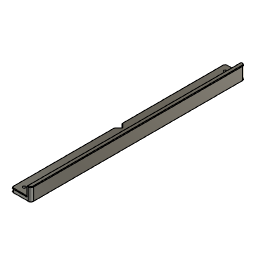
bed_hole_marking_template_x1_Rev2 (Autodesk Fusion 360 design; units mm, degrees)
Autodesk Fusion 360 part; units mm, degrees
sketch "Sketch1" plane through (0, 0, 0) normal (0, 0, 1) x (1, 0, 0) in component "bed_hole_marking_template_x1_Rev2"
  line L0 (7.5, -80) -> (-7.5, -80)
  line L1 (-7.5, -80) -> (-7.5, 80)
  line L2 (-7.5, 80) -> (7.5, 80)
  line L3 (7.5, 80) -> (7.5, -80)
  line L4 (7.5, -80) -> (-7.5, 80) construction
  line L5 (-7.5, -80) -> (7.5, 80) construction
  line L6 (-4.5, -0.0061) -> (-7.5, 2.9939)
  line L7 (0, 0) -> (-10, 0) construction
  circle A0 centre (-2.5, 75) radius 1
  line L8 (-4.5, 0.0061) -> (-7.5, -2.9939)
  line L9 (4.5, 80) -> (4.5, -80)
  circle A1 centre (-2.5, -75) radius 1
  point P0 (-2.5, -75)
  dimension "d1" = 15
  dimension "d2" = 160
  dimension "d3" = 135
  dimension "d4" = 2
  dimension "d5" = 5
  dimension "d6" = 5
  dimension "d7" = 4.5
  dimension "d8" = 3
  constraint horizontal L0
  constraint perpendicular L0 L1
  constraint parallel L0 L2
  constraint parallel L1 L3
  constraint coincident L4 L7.start
  constraint coincident L5 L7.start
  constraint coincident L7.start origin
  constraint coincident L1 L6.end
  constraint horizontal L7
  constraint symmetric L6.start L7 L8.start
  constraint symmetric L6.end L7 L8.end
  constraint symmetric L7 A0.centre P0
  constraint coincident L2 L9.start
  constraint coincident L0 L9.end
  constraint perpendicular L0 L9
  constraint symmetric L7 A0 A1
  measures "d1" distance of L1.end L2.end
  measures "d2" distance of L0.end L1.end
  measures "d3" angle of L6 L7
  measures "d4" diameter of A0
  measures "d5" distance of L1 A0.centre
  measures "d6" distance of L2 A0.centre
  measures "d7" horizontal distance of L7.start L6.start
  measures "d8" distance of L3 L9
extrude "Extrude1" add sketch "Sketch1" against normal blind 3 contours L0 L2 L3 L9 | L0 L1 L2 L6 L8 L9 in component "bed_hole_marking_template_x1_Rev2"
extrude "Extrude2" add sketch "Sketch1" along normal blind 7 contours L0 L2 L3 L9 in component "bed_hole_marking_template_x1_Rev2"
fillet "Fillet1" radius 2 6 edges at (-7.5, 80, -1.5) (7.5, 80, 2) (-7.5, -80, -1.5) (7.5, -80, 2) (-7.5, 2.9939, -1.5) (-7.5, -2.9939, -1.5) in component "bed_hole_marking_template_x1_Rev2"
chamfer "Chamfer1" distance 0.4 angle 45 31 edges at (7.5, 0, 7) (6.9142, -79.4142, 7) (5, -80, 7) (5, 80, 7) (6.9142, 79.4142, 7) (4.5, 0, 7) (-0.5, -80, 0) (-6.9142, -79.4142, 0) (-7.5, -40.9112, 0) (-7.3478, -3.057, 0) (-5.7101, -1.2041, 0) (-7.5, 40.9112, 0) (-7.3478, 3.057, 0) (-5.7101, 1.2041, 0) (-0.5, 80, 0) (-6.9142, 79.4142, 0) (0, 80, -3) (-6.9142, 79.4142, -3) (-7.5, 40.9112, -3) (-7.3478, 3.057, -3) (-5.7101, 1.2041, -3) (-5.7101, -1.2041, -3) (-7.3478, -3.057, -3) (-7.5, -40.9112, -3) (-6.9142, -79.4142, -3) (0, -80, -3) (6.9142, -79.4142, -3) (7.5, 0, -3) (6.9142, 79.4142, -3) (-3.4323, 74.6384, -3) (-3.4323, -75.3616, -3) in component "bed_hole_marking_template_x1_Rev2"
component "bed_hole_marking_template_x1_Rev2" placed x (1, 0, 0) y (0, 1, 0) z (0, 0, 1) at (0, 0, 0)
